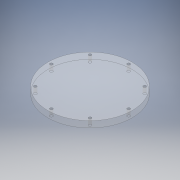
# Autodesk Inventor part: Cover
Saved by Autodesk Inventor 2017 (Build 210142000, 142)
## iProperties
Created: 2016-04-15
Part Number: Cover
Material: Generic
Document SubType Name: Modeling
Designer: Andres
Density: 1 g/cm^3
Appearance: Clear - Light
Mass: 19.88 g
Surface Area: 112.469 cm^2
Volume: 19.88 cm^3
Author: Andres
Autodesk Inventor part; units mm, degrees
ref_plane "YZ Plane" through (0, 0, 0) normal (1, 0, 0) x (0, 1, 0)
ref_plane "XZ Plane" through (0, 0, 0) normal (0, 1, 0) x (-1, 0, 0)
ref_plane "XY Plane" through (0, 0, 0) normal (0, 0, 1) x (1, 0, 0)
sketch "Sketch1" plane through (0, 0, 0) normal (0, 0, 1) x (1, 0, 0)
  circle A0 centre (0, 0) radius 40
  dimension "d47" = 80
  constraints: 1 centre point
  measures "d47" diameter of A0
extrude "Extrusion1" add sketch "Sketch1" along normal blind 6
sketch "Sketch7" plane through (0, 0, 6) normal (0, 0, 1) x (1, 0, 0)
  circle A0 centre (0, 0) radius 40 projected
  circle A1 centre (-36.828, 0) radius 1.5
  circle A2 centre (-26.0413, -26.0413) radius 1.5
  circle A3 centre (0, -36.828) radius 1.5
  circle A4 centre (26.0413, -26.0413) radius 1.5
  circle A5 centre (36.828, 0) radius 1.5
  circle A6 centre (26.0413, 26.0413) radius 1.5
  circle A7 centre (0, 36.828) radius 1.5
  circle A8 centre (-26.0413, 26.0413) radius 1.5
  dimension "d48" = 3
  dimension "d49" = 36.828
  dimension "d52" = 360
  constraints: 8 centre point, 1 horizontal alignment, 17 other
  measures "d48" diameter of A1
  measures "d49" distance of point (0, 0) A1.centre
hole "Hole2" at (-26.0413, 26.0413, 6) at (0, 36.828, 6) at (26.0413, 26.0413, 6) at (36.828, 0, 6) at (26.0413, -26.0413, 6) at (0, -36.828, 6) at (-26.0413, -26.0413, 6) at (-36.828, 0, 6) direction (0, 0, -1) diameter 2.642 end through all thread size "6-32 UNC" class "3B" standard "ANSI Unified Screw Threads"
body "Solid1"
